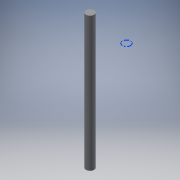
# Autodesk Inventor part: ArmRod
Saved by Autodesk Inventor 2018 (Build 220112000, 112)
## iProperties
Created: 2018-10-19
Part Number: ArmRod
Material: Generic
Document SubType Name: Modeling
Designer: reide
Density: 1 g/cm^3
Appearance: Default
Author: reide
Autodesk Inventor part; units mm, degrees
ref_plane "YZ Plane" through (0, 0, 0) normal (1, 0, 0) x (0, 1, 0)
ref_plane "XZ Plane" through (0, 0, 0) normal (0, 1, 0) x (-1, 0, 0)
sketch "Sketch1" plane through (0, 0, 0) normal (0, 0, 1) x (1, 0, 0)
  circle A0 centre (-3.5783, 0) radius 2.413
  circle A1 centre (-3.5783, 0) radius 2.3
  point P0 (0, 0)
  dimension "d0" = 4.6
  constraints: 2 centre point, 1 coincident
  measures "d0" diameter of A1
ref_plane "Work Plane1" through (-27.3719, -12.081, 76.2) normal (0, 0, -1) x (0, 1, 0)
extrude "Extrusion1" add sketch "Sketch1" along normal up to surface (76.2 mm away) contours A1
body "Solid1"
